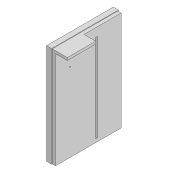
# Autodesk Inventor part: Общий концепт в 3д
Saved by Autodesk Inventor 2022 (Build 260153000, 153)
## iProperties
Created: 2023-02-10
Part Number: Общий концепт в 3д
Material: Типовые
Document SubType Name: Modeling
Designer: Глеб
Density: 1 g/cm^3
Appearance: По умолчанию
Mass: 12000 g
Surface Area: 5800 cm^2
Volume: 12000 cm^3
Author: Глеб
Autodesk Inventor part; units mm, degrees
ref_plane "YZ Plane" through (0, 0, 0) normal (1, 0, 0) x (0, 1, 0)
ref_plane "XZ Plane" through (0, 0, 0) normal (0, 1, 0) x (-1, 0, 0)
ref_plane "XY Plane" through (0, 0, 0) normal (0, 0, 1) x (1, 0, 0)
sketch "Эскиз1" plane through (0, 0, 0) normal (1, 0, 0) x (0, 1, 0)
  line L0 (-270, 200) -> (330, 200)
  line L1 (330, 200) -> (330, -200)
  line L2 (330, -200) -> (-270, -200)
  line L3 (-270, -200) -> (-270, 200)
  line L4 (-270, 200) -> (330, -200) construction
  line L5 (330, 200) -> (-270, -200) construction
  point P0 (30, 0)
  point P1 (0, 0)
  dimension "d0" = 400
  dimension "d1" = 600
  dimension "d73" = 30
  constraints: 12 end point, 2 midpoint, 2 parallel, 1 horizontal, 1 perpendicular
  measures "d0" distance of L0.end L1.end
  measures "d1" distance of L1.end L2.end
  measures "d73" distance of point (30, 0) point (0, 0)
extrude "Выдавливание1" add sketch "Эскиз1" along normal blind 50
sketch "Эскиз3" plane through (50, 0, 0) normal (1, 0, 0) x (0, 0, -1)
  line L0 (-200, 330) -> (-200, -270) projected
  line L1 (-200, -270) -> (200, -270) projected
  line L2 (-200, 330) -> (-196, 330)
  line L3 (-196, 330) -> (-196, -270)
  line L4 (-196, -270) -> (-200, -270)
  line L5 (-200, -270) -> (-200, 330)
  line L6 (200, 330) -> (-200, 330) projected
  line L7 (200, -270) -> (196, -270)
  line L8 (196, -270) -> (196, 330)
  line L9 (196, 330) -> (200, 330)
  line L10 (200, 330) -> (200, -270)
  line L11 (200, -270) -> (200, 330) projected
  line L12 (-200, 330) -> (200, 330)
  line L13 (200, 330) -> (200, 326)
  line L14 (200, 326) -> (-200, 326)
  line L15 (-200, 326) -> (-200, 330)
  point P0 (0, 0)
  point P1 (-196, 326)
  point P2 (196, 326)
  dimension "d74" = 4
  dimension "d75" = 4
  dimension "d76" = 4
  constraints: 24 end point, 6 parallel, 3 horizontal, 3 perpendicular, 3 point on line
  measures "d74" distance between parallel lines of L10 L8
  measures "d75" distance between parallel lines of L0 L3
  measures "d76" distance between parallel lines of L6 L14
extrude "Выдавливание3" cut sketch "Эскиз3" against normal blind 20 contours L2 L3 L14 L0 | L14 L3 L1 L0 | L6 L8 L14 L3 | L6 L10 L14 L8 | L14 L10 L1 L8
sketch "Эскиз4" plane through (50, 0, 0) normal (1, 0, 0) x (0, 0, -1)
  line L0 (68.9117, -237) -> (68.9117, -247) construction
  line L1 (38.9117, -237) -> (38.9117, -247) construction
  line L2 (58.9117, -237) -> (58.9117, -247) construction
  line L3 (58.9117, -237) -> (68.9117, -237) construction
  line L4 (68.9117, -247) -> (58.9117, -247) construction
  line L5 (68.9117, -247) -> (88.9117, -247) construction
  line L6 (88.9117, -237) -> (68.9117, -237) construction
  line L7 (88.9117, -247) -> (88.9117, -237) construction
  line L8 (98.9117, -237) -> (98.9117, -247) construction
  line L9 (88.9117, -237) -> (98.9117, -237) construction
  line L10 (98.9117, -247) -> (88.9117, -247) construction
  line L11 (38.9117, -247) -> (28.9117, -247) construction
  line L12 (28.9117, -237) -> (38.9117, -237) construction
  line L13 (28.9117, -247) -> (28.9117, -237) construction
  line L14 (28.9117, -237) -> (8.9117, -237) construction
  line L15 (28.9117, -247) -> (28.9117, -237) construction
  line L16 (28.9117, -237) -> (8.9117, -237) construction
  line L17 (8.9117, -237) -> (8.9117, -247) construction
  line L18 (8.9117, -247) -> (28.9117, -247) construction
  line L19 (-1.0883, -237) -> (8.9117, -237) construction
  line L20 (-1.0883, -237) -> (-1.0883, -247) construction
  line L21 (8.9117, -247) -> (-1.0883, -247) construction
  line L22 (8.9117, -237) -> (8.9117, -247) construction
  line L23 (53.9117, -250) -> (43.9117, -250)
  line L24 (43.9117, -250) -> (43.9117, 276)
  line L25 (43.9117, 276) -> (53.9117, 276)
  line L26 (53.9117, 276) -> (53.9117, -250)
  line L27 (196, 326) -> (-196, 326) projected
  line L28 (-196, -270) -> (196, -270) projected
  point P0 (0, 0)
  dimension "d80" = 15
  dimension "d81" = 15
  dimension "d82" = 50
  dimension "d83" = 20
  constraints: 8 end point, 2 parallel, 1 horizontal, 1 perpendicular
  measures "d80" distance between parallel lines of L13 L24
  measures "d81" distance between parallel lines of L0 L26
  measures "d82" distance between parallel lines of L27 L25
  measures "d83" distance between parallel lines of L28 L23
extrude "Выдавливание4" cut sketch "Эскиз4" against normal blind 60
sketch "Эскиз5" plane through (50, 0, 0) normal (1, 0, 0) x (0, 0, -1)
  line L0 (-89.8865, 149.6936) -> (-99.7391, 147.983) projected
  line L1 (-99.7391, 147.983) -> (-100.4234, 151.9241) projected
  line L2 (-100.4234, 151.9241) -> (-90.5708, 153.6347) projected
  line L3 (-90.5708, 153.6347) -> (-89.8865, 149.6936) projected
  line L4 (-132.1786, 222.6367) -> (-133.7515, 226.3145) projected
  line L5 (-133.7515, 226.3145) -> (-124.5571, 230.2467) projected
  line L6 (-124.5571, 230.2467) -> (-122.9842, 226.5689) projected
  line L7 (-122.9842, 226.5689) -> (-132.1786, 222.6367) projected
  line L8 (-109.4825, 186.8162) -> (-109.4497, 190.8161) projected
  line L9 (-109.4497, 190.8161) -> (-99.45, 190.734) projected
  line L10 (-99.45, 190.734) -> (-99.4828, 186.7341) projected
  line L11 (-99.4828, 186.7341) -> (-109.4825, 186.8162) projected
  line L12 (-101.3444, 227.5816) -> (-102.6741, 223.8091) projected
  line L13 (-102.6741, 223.8091) -> (-112.1054, 227.1332) projected
  line L14 (-112.1054, 227.1332) -> (-110.7758, 230.9058) projected
  line L15 (-110.7758, 230.9058) -> (-101.3444, 227.5816) projected
  line L16 (-121.5737, 151.067) -> (-130.5132, 155.5487) projected
  line L17 (-130.5132, 155.5487) -> (-128.7205, 159.1245) projected
  line L18 (-128.7205, 159.1245) -> (-119.781, 154.6428) projected
  line L19 (-119.781, 154.6428) -> (-121.5737, 151.067) projected
  line L20 (-73.3529, 162.3525) -> (-66.0686, 169.2037) projected
  line L21 (-66.0686, 169.2037) -> (-63.3281, 166.29) projected
  line L22 (-63.3281, 166.29) -> (-70.6124, 159.4388) projected
  line L23 (-70.6124, 159.4388) -> (-73.3529, 162.3525) projected
  line L24 (-146.4475, 202.9259) -> (-150.1162, 204.5198) projected
  line L25 (-150.1162, 204.5198) -> (-146.1314, 213.6916) projected
  line L26 (-146.1314, 213.6916) -> (-142.4627, 212.0976) projected
  line L27 (-142.4627, 212.0976) -> (-146.4475, 202.9259) projected
  line L28 (-88.6954, 198.226) -> (-94.2983, 189.943) projected
  line L29 (-94.2983, 189.943) -> (-97.6115, 192.1842) projected
  line L30 (-97.6115, 192.1842) -> (-92.0086, 200.4671) projected
  line L31 (-92.0086, 200.4671) -> (-88.6954, 198.226) projected
  line L32 (-87.8306, 208.7569) -> (-91.5842, 207.3746) projected
  line L33 (-91.5842, 207.3746) -> (-95.04, 216.7585) projected
  line L34 (-95.04, 216.7585) -> (-91.2865, 218.1408) projected
  line L35 (-91.2865, 218.1408) -> (-87.8306, 208.7569) projected
  line L36 (-142.6786, 173.9561) -> (-146.3858, 172.4539) projected
  line L37 (-146.3858, 172.4539) -> (-150.1413, 181.7219) projected
  line L38 (-150.1413, 181.7219) -> (-146.434, 183.2241) projected
  line L39 (-146.434, 183.2241) -> (-142.6786, 173.9561) projected
  line L40 (-57.2, 186.602) -> (-55.7515, 196.4965) projected
  line L41 (-55.7515, 196.4965) -> (-51.7937, 195.9171) projected
  line L42 (-51.7937, 195.9171) -> (-53.2422, 186.0226) projected
  line L43 (-53.2422, 186.0226) -> (-57.2, 186.602) projected
  circle A0 centre (-110, 199.3849) radius 60 projected
  point P0 (0, 0)
  constraints: 1 coincident
hole "Отверстие1" at (50, 199.3849, 110) direction (-1, 0, 0) diameter 8.1 depth 80
sketch "Эскиз6" plane through (50, 0, 0) normal (1, 0, 0) x (0, 0, -1)
  line L0 (-196, 326) -> (-196, -270) projected
  line L1 (-196, 326) -> (196, 326)
  line L2 (196, 326) -> (196, 320)
  line L3 (196, 320) -> (-196, 320)
  line L4 (-196, 320) -> (-196, 326)
  point P0 (0, 0)
  dimension "d93" = 6
  dimension "d94" = 392
  constraints: 8 end point, 2 parallel, 1 horizontal, 1 perpendicular
  measures "d93" distance of L1.end L2.end
  measures "d94" distance of L2.end L3.end
extrude "Выдавливание5" add sketch "Эскиз6" along normal blind 70
